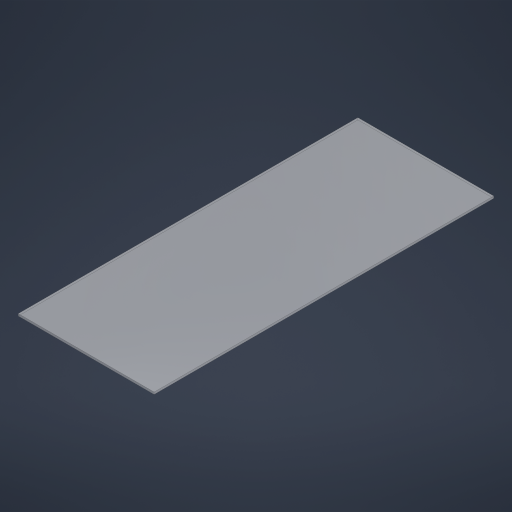
# Autodesk Inventor part: polycarb10x4
Saved by Autodesk Inventor 2023 (Build 270158000, 158)
## iProperties
Created: 2023-01-26
Part Number: polycarb10x4
Material: Polycarbonate, Clear
Document SubType Name: Modeling
Designer: Windows Macbook
Density: 1.2 g/cm^3
Appearance: Polycarbonate - Clear
Author: Windows Macbook
Autodesk Inventor part; units mm, degrees
ref_plane "YZ Plane" through (0, 0, 0) normal (1, 0, 0) x (0, 1, 0)
ref_plane "XZ Plane" through (0, 0, 0) normal (0, 1, 0) x (-1, 0, 0)
ref_plane "XY Plane" through (0, 0, 0) normal (0, 0, 1) x (1, 0, 0)
sketch "Sketch1" plane through (0, 0, 0) normal (0, 1, 0) x (-1, 0, 0)
  line L0 (-50.8, -127) -> (50.8, -127)
  line L1 (50.8, -127) -> (50.8, 127)
  line L2 (50.8, 127) -> (-50.8, 127)
  line L3 (-50.8, 127) -> (-50.8, -127)
  point P0 (0, 0)
  dimension "d0" = 101.6
  dimension "d1" = 254
  constraints: 8 end point, 2 parallel, 1 horizontal, 1 perpendicular
  measures "d0" distance of L2.end L1.end
  measures "d1" distance of L1.end L0.end
extrude "Extrusion1" add sketch "Sketch1" along normal mid plane 1.5875
body "Solid1"
